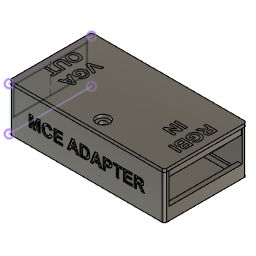
mce_adpater_new_version (Autodesk Fusion 360 design; units mm, degrees)
Autodesk Fusion 360 part; units mm, degrees
note: some values were not read from the file. Chosen so that the rebuilt part matches the saved one: which face or edge a step refers to; the layout of a text. Set by a fixed rule: which sketch regions a step uses.
sketch "스케치1" plane through (0, 0, 0) normal (0, 0, 1) x (1, 0, 0)
  line L0 (0, 0) -> (63.8, 0)
  line L1 (63.8, 0) -> (63.8, 32)
  line L2 (63.8, 32) -> (0, 32)
  line L3 (0, 32) -> (0, 0)
  line L4 (62.8, 1) -> (62.8, 31)
  line L5 (62.8, 31) -> (1, 31)
  line L6 (1, 31) -> (1, 1)
  line L7 (1, 1) -> (62.8, 1)
  line L8 (-2, 34) -> (65.8, 34)
  line L9 (65.8, 34) -> (65.8, -2)
  line L10 (65.8, -2) -> (-2, -2)
  line L11 (-2, -2) -> (-2, 34)
  line L12 (-1, 33) -> (64.8, 33)
  line L13 (64.8, 33) -> (64.8, -1)
  line L14 (64.8, -1) -> (-1, -1)
  line L15 (-1, -1) -> (-1, 33)
  line L16 (0, 30) -> (20.9, 30) construction
  line L17 (37, 0) -> (37, 7)
  line L18 (37, 7) -> (30, 7)
  line L19 (30, 7) -> (30, 0)
  line L20 (27.9, 32) -> (27.9, 25)
  line L21 (27.9, 25) -> (20.9, 25)
  line L22 (20.9, 25) -> (20.9, 32)
  line L23 (30, 7) -> (37, 0) construction
  line L24 (27.9, 25) -> (20.9, 32) construction
  circle A0 centre (24.4, 28.5) radius 1.5
  circle A1 centre (33.5, 3.5) radius 1.5
  line L25 (27.9, 32) -> (27.9, 33)
  line L26 (20.9, 32) -> (20.9, 33)
  line L27 (37, 0) -> (37, -1)
  line L28 (30, 0) -> (30, -1)
  circle A2 centre (24.4, 28.5) radius 2.925
  circle A3 centre (33.5, 3.5) radius 2.925
  dimension "d1" = 63.8
  dimension "d2" = 32
  dimension "d3" = -1
  dimension "d4" = 2
  dimension "d5" = 2
  dimension "d6" = 2
  dimension "d7" = 2
  dimension "d14" = 1
  dimension "d15" = 1
  dimension "d16" = 1
  dimension "d17" = 1
  dimension "d47" = 20.9
  dimension "d48" = 1
  dimension "d49" = 7
  dimension "d50" = 3
  dimension "d51" = 30
  dimension "d58" = 5.85
  constraint horizontal L0
  constraint vertical L1
  constraint horizontal L2
  constraint vertical L3
  constraint coincident L0.start L3.end
  constraint horizontal L8
  constraint vertical L9
  constraint horizontal L10
  constraint vertical L11
  constraint horizontal L12
  constraint vertical L13
  constraint horizontal L14
  constraint vertical L15
  constraint coincident L3 L16.start
  constraint perpendicular L3 L16
  constraint coincident L0 L17.start
  constraint perpendicular L7 L17
  constraint perpendicular L17 L18
  constraint coincident L0 L19.end
  constraint perpendicular L0 L19
  constraint coincident L2 L20.start
  constraint perpendicular L5 L20
  constraint perpendicular L20 L21
  constraint coincident L2 L22.end
  constraint perpendicular L2 L22
  constraint equal L20 L21
  constraint equal L18 L19
  constraint equal L17 L20
  constraint midpoint L24 A0.centre
  constraint midpoint L23 A1.centre
  constraint equal A0 A1
  constraint coincident L16.end L22
  constraint coincident L12 L25.end
  constraint perpendicular L12 L25
  constraint coincident L12 L26.end
  constraint perpendicular L12 L26
  constraint coincident L14 L27.end
  constraint perpendicular L14 L27
  constraint coincident L14 L28.end
  constraint perpendicular L14 L28
  constraint concentric A0 A2
  constraint concentric A1 A3
  constraint equal A2 A3
  measures "d1" distance of L0.start L0.end
  measures "d2" distance of L0.end L1.end
  measures "d4" distance of L0 L10
  measures "d5" distance of L1 L9
  measures "d6" distance of L3 L11
  measures "d7" distance of L2 L8
  measures "d14" distance of L10 L14
  measures "d15" distance of L9 L13
  measures "d16" distance of L8 L12
  measures "d17" distance of L11 L15
  measures "d47" distance of L16.start L16.end
  measures "d48" distance of L5 L16.end
  measures "d49" distance of L20.start L20.end
  measures "d50" diameter of A0
  measures "d51" distance of L3 L19
  measures "d58" diameter of A2
extrude "돌출1" add sketch "스케치1" along normal blind 0.8 contours L7 L17 L18 L19 A3 | L4 L5 L6 L7 L17 L18 L19 L20 L21 L22 | L7 A3 | L5 L20 L21 L22 A2 | L5 A2 | A0 | A1 picked at (33.4626, 1.3347) picked at (24.3626, 30.6653) makes body 1
extrude "돌출2" add sketch "스케치1" along normal blind 3 contours L0 L2 L3 L5 L6 L7 L19 L22 | L0 L7 L17 L19 A3 | L0 L1 L2 L4 L5 L7 L17 L20 | L2 L5 L20 L22 A2 | L7 A3 | L5 A2 picked at (33.1119, 0.9389) picked at (24.3854, 31.1937) bodies 1
extrude "돌출3" add sketch "스케치1" along normal blind 19 contours L0 L2 L3 L12 L14 L15 L26 L28 | L0 L14 L27 L28 | L0 L1 L2 L12 L13 L14 L25 L27 | L2 L12 L25 L26 | L8 L9 L10 L11 bodies 1
extrude "돌출4" cut sketch "스케치1" against normal blind 1.5 from surface at 19 contours L0 L2 L3 L12 L14 L15 L26 L28 | L0 L14 L27 L28 | L0 L1 L2 L12 L13 L14 L25 L27 | L2 L12 L25 L26 bodies 1
sketch "스케치2" plane through (0, 0, 19) normal (0, 0, 1) x (-1, 0, 0)
  line L0 (-64.8, -33) -> (-64.8, 1)
  line L1 (-64.8, 1) -> (1, 1)
  line L2 (1, 1) -> (1, -33)
  line L3 (1, -33) -> (-64.8, -33)
  line L4 (2, 2) -> (-65.8, 2)
  line L5 (-65.8, 2) -> (-65.8, -34)
  line L6 (-65.8, -34) -> (2, -34)
  line L7 (2, -34) -> (2, 2)
  line L8 (2, -34) -> (-65.8, -34)
  line L9 (-65.8, -34) -> (-65.8, 2)
  line L10 (-65.8, 2) -> (2, 2)
  line L11 (2, 2) -> (2, -34)
  constraint horizontal L8
  constraint vertical L9
  constraint horizontal L10
  constraint vertical L11
  constraint coincident L4.end L5.start
  constraint coincident L6.end L7.start
extrude "돌출5" add sketch "스케치2" along normal blind 1.4 separate body contours L0 L1 L2 L3 | L4 L5 L6 L7 L8 L9 L10 L11 makes body 2
extrude "돌출6" add sketch "스케치2" against normal blind 1.5 contours L0 L1 L2 L3 bodies 2
extrude "돌출13" cut sketch "스케치1" along normal through all from surface at 19 contours L7 A3 | L7 A3 bodies 2
sketch "스케치3" plane through (-2, 0, 0) normal (-1, 0, 0) x (0, -1, 0)
  line L0 (-34, 0) -> (2, 0)
  line L1 (2, 0) -> (2, 19)
  line L2 (2, 19) -> (-34, 19)
  line L3 (-34, 19) -> (-34, 0)
  line L4 (-32, 19) -> (0, 19)
  line L5 (0, 19) -> (0, 5.5)
  line L6 (0, 5.5) -> (-32, 5.5)
  line L7 (-32, 5.5) -> (-32, 19)
  line L8 (2, 0) -> (-34, 0)
  line L9 (-16, 19) -> (-16, 5.5) construction
  line L10 (2, 19) -> (-34, 19)
  line L11 (-32, 17.5) -> (0, 17.5)
  dimension "d28" = 5.5
  dimension "d30" = 32
  dimension "d81" = 1.5
  constraint horizontal L4
  constraint vertical L5
  constraint horizontal L6
  constraint vertical L7
  constraint midpoint L4 L9.start
  constraint midpoint L6 L9.end
  constraint symmetric L1 L3 L9
  constraint collinear L4 L10
  constraint coincident L7 L11.start
  constraint coincident L5 L11.end
  constraint perpendicular L5 L11
  measures "d28" distance of L6 L8
  measures "d30" distance of L5.end L6.end
  measures "d81" distance of L4 L11
extrude "돌출7" cut sketch "스케치3" against normal through all contours L2 L4 L5 L7 L10 L11 | L5 L6 L7 L11 bodies 1
extrude "돌출18" add sketch "스케치3" against normal blind 67.6 contours L2 L4 L5 L7 L10 L11 bodies 2
extrude "돌출14" cut sketch "스케치1" along normal through all and the other way through all from surface at 19 contours A1 bodies 2
extrude "돌출12" add sketch "스케치1" against normal blind 1.5 from surface at 17.5 contours L0 L7 L17 L19 A3 | L0 L14 L27 L28 | L7 L17 L18 L19 A3 | L7 A3 | L7 A3 | A1 bodies 1
chamfer "챔퍼1" distance 7 angle 45 1 edges at (33.5, 0, 16) on bodies 1
extrude "돌출15" cut sketch "스케치1" against normal blind 8 from surface at 19 contours L5 A2 | A0 | A1 picked at (24.3626, 30.6653) bodies 1
sketch "스케치4" plane through (64.8, 0, 0) normal (1, 0, 0) x (0, 1, 0)
  line L0 (0, 19) -> (-1, 19)
  line L1 (-1, 17.5) -> (0, 17.5)
  line L2 (32, 17.5) -> (0, 17.5)
  line L3 (0, 17.5) -> (0, 19)
  line L4 (0, 19) -> (32, 19)
  line L5 (32, 19) -> (32, 17.5)
  line L6 (0, 5.5) -> (0, 19)
  line L7 (32, 19) -> (32, 5.5)
  line L8 (-1, 19) -> (-1, 17.5)
  line L9 (33, 17.5) -> (33, 19)
  line L10 (0, 17.5) -> (0, 19)
  line L11 (33, 19) -> (32, 19)
  line L12 (32, 19) -> (32, 17.5)
  line L13 (32, 17.5) -> (33, 17.5)
  constraint horizontal L2
  constraint vertical L3
  constraint horizontal L4
  constraint vertical L5
  constraint coincident L0 L3.end
  constraint coincident L1 L2.start
  constraint collinear L3 L6
  constraint collinear L5 L7
extrude "돌출8" cut sketch "스케치4" against normal blind 10 contours L2 L3 L4 L5 L6 L7 L10 L12 bodies 2
sketch "스케치5" plane through (-1, 0, 0) normal (-1, 0, 0) x (0, -1, 0)
  line L0 (-32, 19) -> (-33, 19)
  line L1 (0, 17.5) -> (1, 17.5)
  line L2 (-32, 19) -> (0, 19)
  line L3 (0, 19) -> (0, 17.5)
  line L4 (0, 17.5) -> (-32, 17.5)
  line L5 (-32, 17.5) -> (-32, 19)
  line L6 (0, 19) -> (0, 5.5)
  line L7 (-32, 5.5) -> (-32, 19)
  line L8 (-33, 19) -> (-33, 17.5)
  line L9 (1, 17.5) -> (1, 19)
  line L10 (0, 19) -> (0, 17.5)
  line L11 (-32, 17.5) -> (-32, 19)
  line L12 (1, 19) -> (0, 19)
  line L13 (-33, 17.5) -> (-32, 17.5)
  constraint horizontal L2
  constraint vertical L3
  constraint horizontal L4
  constraint vertical L5
  constraint coincident L1 L3.end
  constraint coincident L0 L2.start
  constraint collinear L3 L6
  constraint collinear L5 L7
extrude "돌출9" cut sketch "스케치5" against normal blind 10 contours L2 L3 L4 L5 L6 L7 L10 L11 bodies 2
extrude "돌출19" add 2 faces at (-1.3333, 10.6667, 17.5) (65.0667, 21.3333, 17.5) along direction (0, 0, -1) blind 1 on bodies 2 bodies 2
sketch "스케치6" plane through (0, 34, 0) normal (0, 1, 0) x (-1, 0, 0)
  line L0 (-65.8, 0) -> (2, 0)
  line L1 (2, 0) -> (2, 19)
  line L2 (-65.8, 19) -> (-65.8, 0)
  line L3 (-65.8, 4.7) -> (2, 4.7) construction
  line L4 (-29.1, 8.9) -> (-20.9, 8.9)
  line L5 (-20.9, 8.9) -> (-20.9, 4.7)
  line L6 (-20.9, 4.7) -> (-29.1, 4.7)
  line L7 (-29.1, 4.7) -> (-29.1, 8.9)
  line L8 (-29.1, 6.8) -> (-20.9, 6.8) construction
  line L9 (-25, 6.8) -> (-25, 4.7) construction
  line L10 (-28.6, 4.7) -> (-28.6, 6.455)
  line L11 (-28.6, 6.455) -> (-29.1, 6.8)
  line L12 (-21.4, 4.7) -> (-21.4, 6.455)
  line L13 (-21.4, 6.455) -> (-20.9, 6.8)
  line L14 (2, 0) -> (-65.8, 0)
  line L15 (-20.9, 0) -> (-20.9, 4.7) construction
  line L16 (2, 19) -> (-65.8, 19)
  line L17 (2, 5.5) -> (2, 19)
  point P0 (-20.9, 0)
  dimension "d38" = 4.2
  dimension "d39" = 8.2
  dimension "d40" = 2.1
  dimension "d41" = 0.5
  dimension "d42" = 0.345
  dimension "d44" = 4.7
  dimension "d84" = 22.9
  constraint coincident L2 L3.start
  constraint coincident L1 L3.end
  constraint perpendicular L1 L3
  constraint horizontal L4
  constraint vertical L5
  constraint horizontal L6
  constraint vertical L7
  constraint collinear L3 L6
  constraint coincident L7 L8.start
  constraint coincident L5 L8.end
  constraint perpendicular L5 L8
  constraint midpoint L8 L9.start
  constraint midpoint L6 L9.end
  constraint coincident L6 L10.start
  constraint perpendicular L6 L10
  constraint coincident L3 L12.start
  constraint perpendicular L3 L12
  constraint coincident L8.start L11.end
  constraint coincident L8 L13.end
  constraint symmetric L9 L10 L12
  constraint equal L11 L13
  constraint coincident L14 P0
  constraint coincident L3 L5.end
  constraint perpendicular L3 L15
  constraint coincident P0 L15.start
  constraint collinear L5 L15
  measures "d38" distance of L4.end L5.end
  measures "d39" distance of L4.start L4.end
  measures "d40" distance of L4 L8
  measures "d41" distance of L7 L10
  measures "d42" distance of L8 L10.end
  measures "d44" distance of L3 L14
  measures "d84" distance of L5 L17
extrude "돌출10" cut sketch "스케치6" against normal blind 2 contours L4 L5 L6 L7 L10 L11 L12 L13 bodies 1
sketch "스케치7" plane through (0, 0, 19) normal (0, 0, -1) x (1, 0, 0)
  line L0 (-1, 1) -> (64.8, 1)
  line L1 (64.8, 1) -> (64.8, 0)
  line L2 (64.8, -33) -> (-1, -33)
  line L3 (-1, 0) -> (-1, 1)
  line L4 (65.8, 2) -> (-2, 2)
  line L5 (-2, 2) -> (-2, 0)
  line L6 (-2, -34) -> (65.8, -34)
  line L7 (65.8, -34) -> (65.8, 2)
  line L8 (5.5, -0.25) -> (8.5, -0.25)
  line L9 (8.5, -0.25) -> (8.5, -6.75)
  line L10 (8.5, -6.75) -> (5.5, -6.75)
  line L11 (5.5, -6.75) -> (5.5, -0.25)
  line L12 (5.5, -25.25) -> (8.5, -25.25)
  line L13 (8.5, -25.25) -> (8.5, -31.75)
  line L14 (8.5, -31.75) -> (5.5, -31.75)
  line L15 (5.5, -31.75) -> (5.5, -25.25)
  line L16 (55.3, -0.25) -> (58.3, -0.25)
  line L17 (58.3, -0.25) -> (58.3, -6.75)
  line L18 (58.3, -6.75) -> (55.3, -6.75)
  line L19 (55.3, -6.75) -> (55.3, -0.25)
  line L20 (55.3, -25.25) -> (58.3, -25.25)
  line L21 (58.3, -25.25) -> (58.3, -31.75)
  line L22 (58.3, -31.75) -> (55.3, -31.75)
  line L23 (55.3, -31.75) -> (55.3, -25.25)
  line L24 (-2, -16) -> (64.8, -16) construction
  line L25 (5.5, -3.5) -> (8.5, -3.5) construction
  line L26 (5.5, -28.5) -> (8.5, -28.5) construction
  line L27 (55.3, -3.5) -> (58.3, -3.5) construction
  line L28 (64.8, 0) -> (65.6, 0)
  line L29 (-2, 0) -> (-1, 0)
  line L30 (65.6, -32) -> (64.8, -32)
  line L31 (64.8, -32) -> (64.8, -33)
  line L32 (-1, -33) -> (-1, -32)
  line L33 (-1, -32) -> (-2, -32)
  line L34 (-2, -32) -> (-2, -34)
  line L35 (65.6, 0) -> (65.6, -32)
  line L36 (-2, -32) -> (-2, 0)
  line L37 (64.8, 0) -> (64.8, -32)
  dimension "d71" = 3
  dimension "d72" = 7.5
  dimension "d73" = 25
  dimension "d74" = 6.5
  dimension "d75" = 7.5
  constraint horizontal L8
  constraint vertical L9
  constraint horizontal L10
  constraint vertical L11
  constraint horizontal L12
  constraint vertical L13
  constraint horizontal L14
  constraint vertical L15
  constraint horizontal L16
  constraint vertical L17
  constraint horizontal L18
  constraint vertical L19
  constraint horizontal L20
  constraint vertical L21
  constraint horizontal L22
  constraint vertical L23
  constraint equal L8 L12
  constraint equal L9 L13
  constraint equal L8 L16
  constraint equal L9 L17
  constraint equal L8 L20
  constraint equal L9 L21
  constraint symmetric L8 L14 L24
  constraint symmetric L16 L22 L24
  constraint midpoint L11 L25.start
  constraint midpoint L9 L25.end
  constraint midpoint L15 L26.start
  constraint midpoint L13 L26.end
  constraint collinear L9 L13
  constraint collinear L19 L23
  constraint midpoint L19 L27.start
  constraint midpoint L17 L27.end
  constraint collinear L25 L27
  constraint midpoint L24.start L36
  constraint midpoint L24.end L37
  measures "d71" distance of L8.start L8.end
  measures "d72" distance of L5 L11
  measures "d73" distance of L25 L26
  measures "d74" distance of L8.end L9.end
  measures "d75" distance of L7 L17
extrude "돌출16" add sketch "스케치7" along normal blind 10 contours L8 L9 L10 L11 | L12 L13 L14 L15 | L16 L17 L18 L19 | L20 L21 L22 L23 bodies 2
sketch "스케치8" plane through (5.5, 0, 0) normal (-1, 0, 0) x (0, -1, 0)
  line L0 (-6.75, 19) -> (-6.75, 9)
  line L1 (-6.75, 9) -> (-0.25, 9)
  line L2 (-0.25, 9) -> (-0.25, 19)
  circle A0 centre (-3.5, 11.25) radius 1.4
  circle A1 centre (-28.5, 11.25) radius 1.4
  line L3 (-28.5, 11.25) -> (-3.5, 11.25) construction
  line L4 (-3.5, 9) -> (-3.5, 11.25) construction
  line L5 (-25.25, 9) -> (-31.75, 9) construction
  line L6 (-28.5, 9) -> (-28.5, 11.25) construction
  line L7 (-0.25, 19) -> (-6.75, 19)
  point P0 (-25.25, 9)
  point P1 (-31.75, 9)
  dimension "d78" = 2.8
  dimension "d79" = 2.25
  constraint equal A0 A1
  constraint coincident A1.centre L3.start
  constraint coincident A0.centre L3.end
  constraint perpendicular L0 L3
  constraint midpoint L1 L4.start
  constraint coincident A0.centre L4
  constraint horizontal L5
  constraint coincident P0 L5.start
  constraint coincident P1 L5.end
  constraint midpoint L5 L6.start
  constraint perpendicular L3 L6
  constraint coincident L3 A0.centre
  constraint perpendicular L3 L4
  measures "d78" diameter of A0
  measures "d79" distance of L1 A0.centre
extrude "돌출17" cut sketch "스케치8" against normal through all contours A0 | A1 bodies 2
fillet "필렛1" radius 1 8 edges at (65.8, 34, 9.5) (65.8, -2, 9.5) (-2, -2, 9.5) (-2, 34, 9.5) (65.8, 34, 19.7) (65.8, -2, 19.7) (-2, -2, 19.7) (-2, 34, 19.7) on bodies 1 2
sketch "스케치10" plane through (0, 0, 20.4) normal (0, 0, 1) x (-1, 0, 0)
  arc A0 (1, -34) -> (2, -33) centre (1, -33) ccw
  line L0 (2, -33) -> (2, 1)
  arc A1 (2, 1) -> (1, 2) centre (1, 1) ccw
  line L1 (1, 2) -> (-64.8, 2)
  arc A2 (-64.8, 2) -> (-65.8, 1) centre (-64.8, 1) ccw
  line L2 (-65.8, 1) -> (-65.8, -33)
  arc A3 (-65.8, -33) -> (-64.8, -34) centre (-64.8, -33) ccw
  line L3 (-64.8, -34) -> (1, -34)
  circle A4 centre (-33.5, -3.5) radius 2.925
  line L4 (0, -23.5) -> (0, -8.5) construction
  line L5 (0, -8.5) -> (-15, -8.5) construction
  line L6 (-15, -8.5) -> (-15, -23.5) construction
  line L7 (-15, -23.5) -> (0, -23.5) construction
  line L8 (-65.8, -16) -> (2, -16) construction
  line L9 (2, -32) -> (2, 0) construction
  line L10 (-48.8, -26) -> (-48.8, -6) construction
  line L11 (-48.8, -6) -> (-63.8, -6) construction
  line L12 (-63.8, -6) -> (-63.8, -26) construction
  line L13 (-63.8, -26) -> (-48.8, -26) construction
  dimension "d89" = 5
  dimension "d90" = 2
  dimension "d91" = 15
  dimension "d92" = 15
  dimension "d93" = 5
  dimension "d94" = 2
  dimension "d95" = 15
  dimension "d96" = 20
  text T0 "VGA OUT" font "Arial" height 5 bold align centre middle in box 15 x 15 at (0, -23.5) x (0, 1) y (-1, 0) spacing 1
  text T1 "RGBI\nIN" font "Arial" height 5 bold align centre middle in box 20 x 15 at (-48.8, -26) x (0, 1) y (-1, 0) spacing 1
  constraint midpoint L2 L8.start
  constraint midpoint L0 L8.end
  measures "d90" distance of L4 L9
  measures "d94" distance of L2 L12
extrude "돌출20" cut sketch "스케치10" against normal blind 0.0001 text T1 T0 bodies 2
sketch "스케치11" plane through (0, 34, 0) normal (0, 1, 0) x (-1, 0, 0)
  line L0 (-20.9, 6.8) -> (-21.4, 6.455)
  line L1 (-21.4, 6.455) -> (-21.4, 4.7)
  line L2 (-21.4, 4.7) -> (-28.6, 4.7)
  line L3 (-28.6, 4.7) -> (-28.6, 6.455)
  line L4 (-28.6, 6.455) -> (-29.1, 6.8)
  line L5 (-29.1, 6.8) -> (-29.1, 8.9)
  line L6 (-29.1, 8.9) -> (-20.9, 8.9)
  line L7 (-20.9, 8.9) -> (-20.9, 6.8)
  line L8 (1, 0) -> (1, 19)
  line L9 (1, 19) -> (-64.8, 19)
  line L10 (-64.8, 19) -> (-64.8, 0)
  line L11 (-64.8, 0) -> (1, 0)
  line L12 (-25, 8.9) -> (-25, 4.7) construction
  line L13 (-31, 10.9) -> (-19, 10.9) construction
  line L14 (-19, 10.9) -> (-19, 14.9) construction
  line L15 (-19, 14.9) -> (-31, 14.9) construction
  line L16 (-31, 14.9) -> (-31, 10.9) construction
  dimension "d99" = 4
  dimension "d100" = 2
  dimension "d101" = 4
  dimension "d102" = 12
  text T0 "USB" font "Arial" height 4 bold align centre middle in box 12 x 4 at (-31, 10.9) x (1, 0) y (0, 1) spacing 1
  constraint midpoint L6 L12.start
  constraint midpoint L2 L12.end
  measures "d100" distance of L6 L13
extrude "돌출21" cut sketch "스케치11" against normal blind 0.5 text T0 bodies 1
sketch "스케치12" plane through (0, -2, 0) normal (0, -1, 0) x (1, 0, 0)
  line L0 (-1, 19) -> (-1, 0)
  line L1 (-1, 0) -> (64.8, 0)
  line L2 (64.8, 0) -> (64.8, 19)
  line L3 (64.8, 19) -> (-1, 19)
  line L4 (2, 4.5) -> (61.8, 4.5) construction
  line L5 (61.8, 4.5) -> (61.8, 14.5) construction
  line L6 (61.8, 14.5) -> (2, 14.5) construction
  line L7 (2, 14.5) -> (2, 4.5) construction
  line L8 (-1, 9.5) -> (64.8, 9.5) construction
  dimension "d105" = 5
  dimension "d106" = 3
  dimension "d107" = 3
  dimension "d108" = 10
  text T0 "MCE ADAPTER" font "Arial" height 5 bold align centre middle in box 59.8 x 10 at (2, 4.5) x (1, 0) y (0, 1) spacing 1 kerned
  constraint midpoint L0 L8.start
  constraint midpoint L2 L8.end
  measures "d106" distance of L2 L5
  measures "d107" distance of L0 L7
extrude "돌출22" cut sketch "스케치12" against normal blind 0.5 text T0 bodies 1
chamfer "챔퍼2" distance 1 angle 45 1 edges at (25, 32, 8.9) on bodies 1
fillet "필렛2" radius 0.5 8 edges at (29.1, 33.5, 8.9) (29.1, 33, 6.8) (28.6, 33, 6.455) (20.9, 33.5, 8.9) (20.9, 33, 6.8) (28.6, 33, 4.7) (21.4, 33, 4.7) (21.4, 33, 6.455) on bodies 1
sketch "스케치13" plane through (0, 0, 0) normal (0, 0, 1) x (1, 0, 0)
extrude "돌출28" cut 2 faces at (65.3333, 0, 17.6667) (-1.6667, 0, 17.6667) along direction (0, 1, 0) blind 0.16 on bodies 2 bodies 2
extrude "돌출29" cut 2 faces at (-1.6667, 32, 17.6667) (65.3333, 32, 17.6667) along direction (0, -1, 0) blind 0.16 on bodies 2 bodies 2
extrude "돌출30" cut 1 faces at (20.9333, 33, 18.5) along direction (0, -1, 0) blind 0.16 on bodies 2 bodies 2
extrude "돌출31" cut 1 faces at (42.8667, -1, 18.5) along direction (0, 1, 0) blind 0.16 on bodies 2 bodies 2
extrude "돌출32" cut 2 faces at (-1, -0.56, 18.5) (-1, 32.28, 18.5) along direction (1, 0, 0) blind 0.16 on bodies 2 bodies 2
extrude "돌출33" cut 2 faces at (64.8, 32.56, 18.5) (64.8, -0.28, 18.5) along direction (-1, 0, 0) blind 0.16 on bodies 2 bodies 2
equation "d4 = WALL_WIDTH"
equation "d5 = WALL_WIDTH"
equation "d6 = WALL_WIDTH"
equation "d7 = WALL_WIDTH"
equation "d10 = PCB_MOUNT"
equation "d12 = WALL_HEIGHT"
equation "d14 = WALL_WIDTH / 2"
equation "d15 = WALL_WIDTH / 2"
equation "d16 = WALL_WIDTH / 2"
equation "d17 = WALL_WIDTH / 2"
equation "WALL_WIDTH = 2 mm"
equation "WALL_HEIGHT = 19 mm"
equation "d20 = WALL_HEIGHT"
equation "d21 = -JUNCTION"
equation "d25 = -JUNCTION"
equation "PCB_MOUNT = 3 mm"
equation "d28 = PCB_MOUNT + 2.5 mm"
equation "JUNCTION = 1.5 mm"
equation "CONNECTOR_DEPTH = 10 mm"
equation "d34 = -CONNECTOR_DEPTH"
equation "d36 = -CONNECTOR_DEPTH"
equation "d44 = PCB_MOUNT + 1.7 mm"
equation "d45 = -WALL_WIDTH"
equation "d49 = HOLE_SIZE"
equation "d55 = WALL_HEIGHT - JUNCTION"
equation "d59 = WALL_HEIGHT"
equation "d62 = WALL_HEIGHT"
equation "d65 = HOLE_SIZE"
equation "HOLE_SIZE = 7 mm"
equation "d68 = WALL_HEIGHT"
equation "d69 = -HOLE_SIZE - 1 mm"
equation "tolerance = 0.16 mm"
equation "d125 = -tolerance"
equation "d127 = -tolerance"
equation "d129 = -tolerance"
equation "d131 = -tolerance"
equation "d133 = -tolerance"
equation "d135 = -tolerance"
named bodies: "Base", "Lid"
